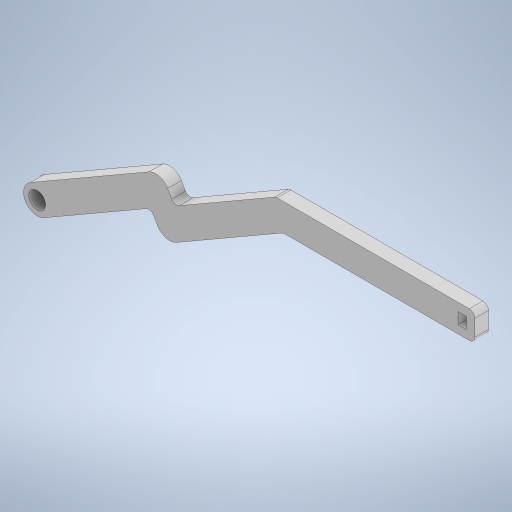
# Autodesk Inventor part: 茎固定パーツ
Saved by Autodesk Inventor 2024.3 (Build 283343000, 343)
## iProperties
Created: 2024-10-08
Part Number: 茎固定パーツ
Material: 一般
Document SubType Name: Modeling
Designer: hikou
Density: 1 g/cm^3
Appearance: 既定
Author: hikou
Autodesk Inventor part; units mm, degrees
ref_plane "YZ Plane" through (0, 0, 0) normal (1, 0, 0) x (0, 1, 0)
ref_plane "XZ Plane" through (0, 0, 0) normal (0, 1, 0) x (-1, 0, 0)
ref_plane "XY Plane" through (0, 0, 0) normal (0, 0, 1) x (1, 0, 0)
sketch "スケッチ1" plane through (0, 0, 0) normal (0, 0, 1) x (1, 0, 0)
  line L0 (0, 0) -> (72.6795, 0)
  line L1 (2.6795, -10) -> (72.6795, -10)
  line L2 (72.6795, 0) -> (72.6795, -10)
  line L3 (2.6795, -10) -> (-83.923, -60)
  line L4 (-36.9615, -21.3397) -> (0, 0)
  line L5 (-83.923, -60) -> (-93.923, -42.6795)
  line L6 (-93.923, -42.6795) -> (-85.2628, -37.6795)
  line L7 (-85.2628, -37.6795) -> (-41.9615, -12.6795)
  line L8 (-41.9615, -12.6795) -> (-36.9615, -21.3397)
  line L9 (-88.923, -51.3397) -> (-45.6218, -26.3397)
  line L10 (-45.6218, -26.3397) -> (-40.6218, -35)
  dimension "d1" = 70
  dimension "d2" = 10
  dimension "d3" = 100
  dimension "d4" = 150
  dimension "d5" = 10
  dimension "d6" = 20
  dimension "d42" = 60
  dimension "d43" = 50
  dimension "d44" = 10
  constraints: 22 end point, 3 perpendicular, 2 horizontal, 2 midpoint, 1 coincident, 1 parallel
  measures "d1" distance of L1.start L1.end
  measures "d2" distance of L0.end L1.end
  measures "d3" distance of L1.start L3.end
  measures "d4" angle of L1 L3
  measures "d5" distance between parallel lines of L4 L3
  measures "d6" distance of L3.end L5.end
  measures "d42" distance between parallel lines of L5 L8
  measures "d43" distance of L9.start L9.end
  measures "d44" distance of L9.end L10.end
extrude "押し出し1" add sketch "スケッチ1" along normal mid plane 5 contours L0 L2 L1 L3 L10 L9 L5 L6 L7 L8 L4
sketch "スケッチ2" plane through (0, 0, 2.5) normal (0, 0, 1) x (1, 0, 0)
  line L0 (66.5795, -7.05) -> (69.6795, -7.05)
  line L1 (69.6795, -7.05) -> (69.6795, -2.95)
  line L2 (69.6795, -2.95) -> (66.5795, -2.95)
  line L3 (66.5795, -2.95) -> (66.5795, -7.05)
  line L4 (66.5795, -7.05) -> (69.6795, -2.95) construction
  line L5 (69.6795, -7.05) -> (66.5795, -2.95) construction
  line L6 (72.6795, 0) -> (0, 0) projected
  line L7 (2.6795, -10) -> (72.6795, -10) projected
  line L8 (72.6795, -10) -> (72.6795, 0) projected
  point P0 (68.1295, -5)
  dimension "d12" = 2.95
  dimension "d13" = 2.95
  dimension "d14" = 3
  dimension "d15" = 3.1
  constraints: 12 end point, 2 midpoint, 2 parallel, 1 horizontal, 1 perpendicular
  measures "d12" distance between parallel lines of L2 L6
  measures "d13" distance between parallel lines of L7 L0
  measures "d14" distance between parallel lines of L8 L1
  measures "d15" distance between parallel lines of L1 L3
extrude "押し出し2" cut sketch "スケッチ2" against normal blind 5
sketch "スケッチ5" plane through (0, 0, 2.5) normal (0, 0, 1) x (1, 0, 0)
  line L0 (-41.9615, -12.6795) -> (-93.923, -42.6795) projected
  line L1 (-93.923, -42.6795) -> (-88.923, -51.3397) projected
  circle A0 centre (-87.0929, -44.5096) radius 3.05
  point P0 (0, 0)
  dimension "d45" = 5
  dimension "d46" = 5
  dimension "d47" = 6.1
  constraints: 1 centre point, 1 coincident
  measures "d45" distance from line of L0 point (-87.093, -44.51)
  measures "d46" distance from line of L1 point (-87.093, -44.51)
  measures "d47" diameter of A0
hole "穴3" at (-87.0929, -44.5096, 2.5) direction (0, 0, -1) diameter 6.1 end through all
fillet "フィレット2" radius 2 10 edges at (-93.923, -42.6795, 0) (-88.923, -51.3397, 0) (-41.9615, -12.6795, 0) (-36.9615, -21.3397, 0) (-40.6218, -35, 0) (-45.6218, -26.3397, 0) (2.6795, -10, 0) (0, 0, 0) (72.6795, 0, 0) (72.6795, -10, 0)
sketch "スケッチ6" plane through (0, 0, 2.5) normal (0, 0, 1) x (1, 0, 0)
  arc A0 (70.6795, -10) -> (72.6795, -8) centre (70.6795, -8) ccw projected
  line L0 (72.6795, -8) -> (72.6795, -2) projected
  arc A1 (72.6795, -2) -> (70.6795, 0) centre (70.6795, -2) ccw projected
  line L1 (70.6795, 0) -> (0.5359, 0) projected
  arc A2 (0.5359, 0) -> (-0.4641, -0.2679) centre (0.5359, -2) ccw projected
  line L2 (-0.4641, -0.2679) -> (-35.2295, -20.3397) projected
  arc A3 (-37.9615, -19.6077) -> (-35.2295, -20.3397) centre (-36.2295, -18.6077) ccw projected
  line L3 (-37.9615, -19.6077) -> (-40.9615, -14.4115) projected
  arc A4 (-40.9615, -14.4115) -> (-43.6936, -13.6795) centre (-42.6936, -15.4115) ccw projected
  line L4 (-43.6936, -13.6795) -> (-92.191, -41.6795) projected
  arc A5 (-92.191, -41.6795) -> (-92.923, -44.4115) centre (-91.191, -43.4115) ccw projected
  line L5 (-92.923, -44.4115) -> (-89.923, -49.6077) projected
  arc A6 (-89.923, -49.6077) -> (-87.191, -50.3397) centre (-88.191, -48.6077) ccw projected
  line L6 (-87.191, -50.3397) -> (-47.3538, -27.3397) projected
  arc A7 (-44.6218, -28.0718) -> (-47.3538, -27.3397) centre (-46.3538, -29.0718) ccw projected
  line L7 (-44.6218, -28.0718) -> (-41.6218, -33.2679) projected
  arc A8 (-41.6218, -33.2679) -> (-38.8897, -34) centre (-39.8897, -32.2679) ccw projected
  line L8 (-38.8897, -34) -> (2.2154, -10.2679) projected
  arc A9 (3.2154, -10) -> (2.2154, -10.2679) centre (3.2154, -12) ccw projected
  line L9 (3.2154, -10) -> (70.6795, -10) projected
  circle A10 centre (-87.0929, -44.5096) radius 3.05 projected
  line L10 (66.5795, -2.95) -> (69.6795, -2.95) projected
  line L11 (69.6795, -2.95) -> (69.6795, -7.05) projected
  line L12 (69.6795, -7.05) -> (66.5795, -7.05) projected
  line L13 (66.5795, -7.05) -> (66.5795, -2.95) projected
  circle A11 centre (-87.0929, -44.5096) radius 5
  point P0 (0, 0)
  point P1 (-84.5929, -48.8397)
  point P2 (-91.423, -47.0096)
  point P3 (-89.5929, -40.1795)
  constraints: 1 centre point, 1 coincident, 1 tangent
extrude "押し出し3" cut sketch "スケッチ6" against normal blind 10 contours L6 A6 L5 A11 | L5 A5 L4 A11
sketch "スケッチ7" plane through (0, 0, 2.5) normal (0, 0, 1) x (1, 0, 0)
  line L0 (-43.6936, -13.6795) -> (-89.5929, -40.1795) projected
  line L1 (-37.9615, -19.6077) -> (-40.9615, -14.4115) projected
  line L2 (-38.8897, -34) -> (2.2154, -10.2679) projected
  line L3 (-44.6218, -28.0718) -> (-41.6218, -33.2679) projected
  circle A0 centre (-43.7917, -19.5096) radius 5
  circle A1 centre (-38.7917, -28.1699) radius 5
  line L4 (66.5795, -2.95) -> (69.6795, -2.95) projected
  line L5 (69.6795, -2.95) -> (69.6795, -7.05) projected
  line L6 (69.6795, -7.05) -> (66.5795, -7.05) projected
  line L7 (66.5795, -7.05) -> (66.5795, -2.95) projected
  circle A2 centre (-87.0929, -44.5096) radius 3.05 projected
  arc A3 (-89.5929, -40.1795) -> (-84.5929, -48.8397) centre (-87.0929, -44.5096) ccw projected
  line L8 (-84.5929, -48.8397) -> (-47.3538, -27.3397) projected
  arc A4 (-44.6218, -28.0718) -> (-47.3538, -27.3397) centre (-46.3538, -29.0718) ccw projected
  line L9 (-44.6218, -28.0718) -> (-41.6218, -33.2679) projected
  arc A5 (-41.6218, -33.2679) -> (-38.8897, -34) centre (-39.8897, -32.2679) ccw projected
  line L10 (-38.8897, -34) -> (2.2154, -10.2679) projected
  arc A6 (3.2154, -10) -> (2.2154, -10.2679) centre (3.2154, -12) ccw projected
  line L11 (3.2154, -10) -> (70.6795, -10) projected
  arc A7 (70.6795, -10) -> (72.6795, -8) centre (70.6795, -8) ccw projected
  line L12 (72.6795, -8) -> (72.6795, -2) projected
  arc A8 (72.6795, -2) -> (70.6795, 0) centre (70.6795, -2) ccw projected
  line L13 (70.6795, 0) -> (0.5359, 0) projected
  arc A9 (0.5359, 0) -> (-0.4641, -0.2679) centre (0.5359, -2) ccw projected
  line L14 (-0.4641, -0.2679) -> (-35.2295, -20.3397) projected
  arc A10 (-37.9615, -19.6077) -> (-35.2295, -20.3397) centre (-36.2295, -18.6077) ccw projected
  line L15 (-37.9615, -19.6077) -> (-40.9615, -14.4115) projected
  arc A11 (-40.9615, -14.4115) -> (-43.6936, -13.6795) centre (-42.6936, -15.4115) ccw projected
  line L16 (-43.6936, -13.6795) -> (-89.5929, -40.1795) projected
  point P0 (0, 0)
  point P1 (-36.2917, -32.5)
  point P2 (-43.1218, -30.6699)
  point P3 (-46.2917, -15.1795)
  point P4 (-39.4615, -17.0096)
  dimension "d58" = 5
  dimension "d59" = 5
  dimension "d60" = 5
  dimension "d61" = 5
  constraints: 2 centre point, 2 coincident
  measures "d58" distance from line of L0 point (-43.792, -19.51)
  measures "d59" distance from line of L1 point (-43.792, -19.51)
  measures "d60" distance from line of L2 point (-38.792, -28.17)
  measures "d61" distance from line of L3 point (-38.792, -28.17)
extrude "押し出し4" cut sketch "スケッチ7" against normal blind 10 contours A11 L1 A0 L0 | A1 L2 A5 L3
equation "\"d12\" = d13"
equation "\"d46\" = d45"
equation "\"d59\" = d58"
equation "\"d60\" = d58"
equation "\"d61\" = d58"
